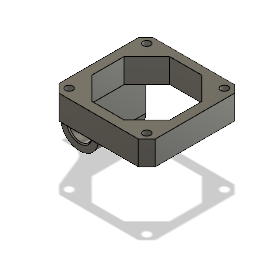
dial_indicator_fan_mount (Autodesk Fusion 360 design; units mm, degrees)
Autodesk Fusion 360 part; units mm, degrees
sketch "Sketch1" plane through (0, 0, 0) normal (0, 0, 1) x (1, 0, 0)
  line L0 (0, 0) -> (39.75, 0)
  line L1 (39.75, 0) -> (39.75, 39.75)
  line L2 (39.75, 39.75) -> (0, 39.75)
  line L3 (0, 39.75) -> (0, 0)
  line L4 (3.875, 35.875) -> (35.875, 35.875) construction
  line L5 (35.875, 35.875) -> (35.875, 3.875) construction
  line L6 (35.875, 3.875) -> (3.875, 3.875) construction
  line L7 (3.875, 3.875) -> (3.875, 35.875) construction
  line L8 (3.875, 19.875) -> (0, 19.875) construction
  line L9 (19.875, 35.875) -> (19.875, 39.75) construction
  circle A0 centre (3.875, 35.875) radius 1.55
  circle A1 centre (35.875, 35.875) radius 1.55
  circle A2 centre (35.875, 3.875) radius 1.55
  circle A3 centre (3.875, 3.875) radius 1.55
  line L10 (19.875, 35.875) -> (19.875, 19.875) construction
  line L11 (19.875, 19.875) -> (3.875, 19.875) construction
  line L12 (35.875, 26.5024) -> (26.5024, 35.875)
  line L13 (26.5024, 35.875) -> (13.2476, 35.875)
  line L14 (13.2476, 35.875) -> (3.875, 26.5024)
  line L15 (3.875, 26.5024) -> (3.875, 13.2476)
  line L16 (3.875, 13.2476) -> (13.2476, 3.875)
  line L17 (13.2476, 3.875) -> (26.5024, 3.875)
  line L18 (26.5024, 3.875) -> (35.875, 13.2476)
  line L19 (35.875, 13.2476) -> (35.875, 26.5024)
  dimension "d1" = 39.75
  dimension "d2" = 39.75
  dimension "d3" = 32
  dimension "d4" = 32
  dimension "d5" = 3.1
  measures "d1" distance of L1 L3
  measures "d3" distance of L0.start
  measures "d5" diameter of A1
extrude "Extrude1" add sketch "Sketch1" along normal blind 10 makes body 1
sketch "Sketch2" plane through (0, 0, 0) normal (0, -1, 0) x (1, 0, 0)
  line L0 (0, 0) -> (39.75, 0)
  line L1 (39.75, 0) -> (39.75, 10)
  line L2 (39.75, 10) -> (0, 10)
  line L3 (0, 10) -> (0, 0)
  circle A0 centre (47.5, 28.335) radius 4.8
  line L4 (39.75, 5) -> (55.25, 5)
  line L5 (47.5, 28.335) -> (47.5, 5) construction
  line L6 (55.25, 5) -> (55.25, 36.135)
  line L7 (55.25, 36.135) -> (39.75, 36.135)
  line L8 (39.75, 36.135) -> (39.75, 10)
  line L9 (47.5, 33.135) -> (47.5, 36.135) construction
  dimension "d9" = 9.6
  dimension "d10" = 15.5
  dimension "d11" = 23.335
  dimension "d13" = 3
  measures "d9" diameter of A0
  measures "d11" distance of L0.start
extrude "Extrude2" add sketch "Sketch2" against normal blind 20 contours L1 L4 L6 L7 L8 bodies 1
fillet "Fillet1" radius 7.5 2 edges at (39.75, 10, 36.135) (55.25, 10, 36.135) on bodies 1
chamfer "Chamfer1" distance 3.5 angle 45 4 edges at (39.75, 39.75, 5) (39.75, 0, 2.5) (0, 39.75, 5) (0, 0, 5) on bodies 1
chamfer "Chamfer2" distance 0.4 angle 45 10 edges at (43.0248, 0, 30.0708) (55.25, 0, 16.8175) (53.0533, 0, 33.9383) (47.5, 0, 36.135) (41.9467, 0, 33.9383) (39.75, 0, 19.3175) (45.75, 0, 5) (19.875, 0, 0) (21.625, 0, 10) (43.0248, 20, 26.5992) on bodies 1
chamfer "Chamfer4" distance 14 angle 45 1 edges at (55.25, 10.2, 5) on bodies 1
fillet "Fillet3" radius 2.5 2 edges at (55.25, 10.2, 19) (41.25, 10.2, 5) on bodies 1
chamfer "Chamfer5" distance 16.25 distance2 6.4999 1 edges at (39.75, 20, 7.5) measured on face at (39.75, 30.8333, 5) on bodies 1
chamfer "Chamfer6" distance 10 distance2 16.1 1 edges at (43, 20, 10) measured on face at (49.5517, 20, 17.1391) on bodies 1
fillet "Fillet6" radius 6 2 edges at (46.2499, 20, 15) (42.9999, 20, 20) on bodies 1
move_body "Move1" bodies 1 to x (1, 0, 0) y (0, 0, 1) z (0, -1, 0) at (0, 0, 0)
mirror "Mirror1" about plane through (0, 0, 39.75) normal (-1, 0, 0) of bodies 1 makes body 2
hidden bodies 1
equation "d11 = 18.55 mm + ( 9.57 / 2 ) * 1 mm"
